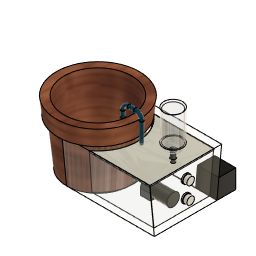
양액 만드는 화분 (Autodesk Fusion 360 design; units mm, degrees)
Autodesk Fusion 360 part; units mm, degrees
note: some values were not read from the file. Chosen so that the rebuilt part matches the saved one: which bodies a step acts on; which sketch regions a step uses; which face or edge a step refers to.
sketch "스케치1" plane through (0, 0, 0) normal (0, 0, 1) x (1, 0, 0)
  circle A0 through (55, 25, 50) (10, 50.9808, 50) (10, -0.9808, 50)
  circle A1 centre (25, 25) radius 25
sketch "스케치1 (curves 50 mm off its plane)" plane through (0, 0, 50) normal (0, 0, 1) x (1, 0, 0)
  circle A0 centre (25, 25) radius 30
loft "로프트1" add profiles "스케치1", "스케치1 (curves 50 mm off its plane)" section 1 section 2 makes body 1
shell "쉘1" thickness 3 removed faces 1 at (36.9822, 20.8839, 50) on bodies 1
sketch "스케치2" plane through (0, 0, 50) normal (0, 0, 1) x (-1, 0, 0)
  circle A0 centre (-25, -25) radius 26.985
  circle A1 centre (-25, -25) radius 30
  circle A2 centre (-25, -25) radius 33
  dimension "d2" = 3
sketch "스케치3" plane through (0, 0, 0) normal (0, 0, -1) x (1, 0, 0)
  circle A0 centre (25, -25) radius 25
  circle A1 centre (25, -25) radius 28
  dimension "d3" = 3
loft "로프트2" add profiles "스케치3", "스케치2" section 1 contours A0 | A1 section 2 contours A2 separate body makes body 2
shell "쉘2" thickness 3 removed faces 1 at (19.7673, 16.6449, 50) on bodies 2
sketch "스케치4" plane through (0, 0, 0) normal (0, 1, 0) x (1, 0, 0)
  line L0 (-8, -37) -> (-8, 0)
  line L1 (-8, -37) -> (58, -37)
  line L2 (58, -37) -> (58, 0)
  line L3 (58, 0) -> (-8, 0)
  constraint vertical L0
  constraint perpendicular L0 L1
  constraint perpendicular L1 L2
  constraint perpendicular L0 L3
extrude "돌출1" cut sketch "스케치4" along normal blind 75 and the other way blind 20 bodies 2
combine "결합1" operation add target body 1 tool bodies 2
sketch "스케치5" plane through (0, 0, 0) normal (0, 0, -1) x (1, 0, 0)
  circle A0 centre (25, -25) radius 25
  line L0 (25, 0) -> (95, 0)
  line L1 (95, 0) -> (95, -50)
  line L2 (95, -50) -> (25, -50)
  constraint coincident A0 L0.start
  constraint tangent A0 L0
  constraint horizontal L0
  constraint perpendicular L0 L1
  constraint coincident A0 L2.end
  constraint tangent A0 L2
  constraint perpendicular L1 L2
sketch "스케치6" plane through (0, 0, 50) normal (0, 0, 1) x (-1, 0, 0)
  circle A0 centre (-25, -25) radius 33
  circle A1 centre (-25, -25) radius 26.985
  line L0 (-25, -55) -> (-95, -55)
  line L1 (-95, -55) -> (-95, 5)
  line L2 (-95, 5) -> (-25, 5)
  circle A2 centre (-25, -25) radius 30
  constraint horizontal L0
  constraint perpendicular L0 L1
  constraint perpendicular L1 L2
  constraint concentric A0 A2
loft "로프트3" add profiles "스케치5", "스케치6" section 1 contours A0 L0 L1 L2 section 2 contours A0 L0 L2 A2 | A0 L0 L1 L2 picked at (-55.9441, -25) separate body makes body 3
sketch "스케치7" plane through (0, 0, 0) normal (0, 1, 0) x (1, 0, 0)
  line L0 (95, -50) -> (95, -37)
  line L1 (95, -37) -> (25, -37)
  line L2 (25, -37) -> (25, -50)
  line L3 (25, -50) -> (95, -50)
  constraint vertical L0
  constraint perpendicular L0 L1
  constraint perpendicular L1 L2
  constraint perpendicular L0 L3
extrude "돌출2" cut sketch "스케치7" along normal mid plane 210 bodies 3
shell "쉘3" thickness 3 removed faces 1 at (81.2007, 24.21, 37) on bodies 3
sketch "스케치8" plane through (0, 0, 3) normal (0, 0, 1) x (-1, 0, 0)
  line L0 (-92, -2.715) -> (-92, -47.285)
  line L1 (-92, -47.285) -> (-42.4675, -47.285)
  arc A0 (-42.4675, -2.715) -> (-42.4675, -47.285) centre (-25, -25) ccw
  line L2 (-42.4675, -2.715) -> (-92, -2.715)
sketch "스케치9" plane through (0, 0, 37) normal (0, 0, 1) x (-1, 0, 0)
  arc A0 (-43.6042, 0.685) -> (-43.6042, -50.685) centre (-25, -25) ccw
  line L0 (-43.6042, -50.685) -> (-92, -50.685)
  line L1 (-92, -50.685) -> (-92, 0.685)
  line L2 (-92, 0.685) -> (-43.6042, 0.685)
  line L3 (-25, 3.7) -> (-95, 3.7)
  line L4 (-95, 3.7) -> (-95, -53.7)
  line L5 (-95, -53.7) -> (-25, -53.7)
  arc A1 (-25, 3.7) -> (-25, -53.7) centre (-25, -25) ccw
loft "로프트4" add profiles "스케치8", "스케치9" section 1 section 2 contours A0 L0 L1 L2 separate body makes body 4
sketch "스케치10" plane through (0, 0, 0) normal (0, 1, 0) x (1, 0, 0)
  line L0 (92, -34) -> (92, -3)
  line L1 (92, -34) -> (43, -34)
  line L2 (43, -34) -> (41, -3)
  line L3 (41, -3) -> (92, -3)
  constraint vertical L0
  constraint perpendicular L0 L1
  constraint perpendicular L0 L3
extrude "돌출3" cut sketch "스케치10" along normal mid plane 180 bodies 4
combine "결합2" operation add target body 3 tool bodies 4
sketch "스케치11" plane through (0, 0, 37) normal (0, 0, 1) x (-1, 0, 0)
  line L0 (-25, 3.7) -> (-95, 3.7)
  line L1 (-95, 3.7) -> (-95, -53.7)
  line L2 (-95, -53.7) -> (-25, -53.7)
  arc A0 (-25, 3.7) -> (-25, -53.7) centre (-25, -25) ccw
  circle A1 centre (-85, -25) radius 1.5
  dimension "d58" = 3
  measures "d58" diameter of A1
extrude "돌출4" cut sketch "스케치11" against normal blind 6 contours A1 bodies 3
sketch "스케치12" plane through (0, 0, 37) normal (0, 0, 1) x (-1, 0, 0)
  circle A0 centre (-85, -25) radius 1.5
  line L0 (-25, 3.7) -> (-95, 3.7)
  line L1 (-95, 3.7) -> (-95, -53.7)
  line L2 (-95, -53.7) -> (-25, -53.7)
  arc A1 (-25, 3.7) -> (-25, -53.7) centre (-25, -25) ccw
  circle A2 centre (-85, -25) radius 2.5
  dimension "d59" = 5
  constraint concentric A0 A2
  measures "d59" diameter of A2
extrude "돌출5" add sketch "스케치12" against normal blind 3 separate body contours A0 makes body 5
extrude "돌출6" add sketch "스케치12" along normal blind 15 contours A0 | A2 bodies 5
sketch "스케치13" plane through (0, 0, 52) normal (0, 0, 1) x (-1, 0, 0)
  circle A0 centre (-85, -25) radius 2.5
  circle A1 centre (-85, -25) radius 7.5
  constraint concentric A0 A1
extrude "돌출7" add sketch "스케치13" along normal blind 30 separate body contours A0 | A1 makes body 6
fillet "모깎기1" radius 4 1 edges at (91.9925, 27.7121, 52) on bodies 6
sketch "스케치14" plane through (0, 0, 0) normal (1, 0, 0) x (0, 1, 0)
  circle A0 centre (25, 10.5) radius 7.5
  line L0 (32.5, 10.5) -> (32.5, 3)
  line L1 (17.5, 10.5) -> (17.5, 3)
  line L2 (17.5, 3) -> (32.5, 3)
  constraint coincident A0 L0.start
  constraint tangent A0 L0
  constraint vertical L0
  constraint coincident A0 L1.start
  constraint tangent A0 L1
  constraint vertical L1
  constraint perpendicular L0 L2
extrude "돌출8" add sketch "스케치14" along normal blind 92 and the other way blind -62 separate body makes body 7
extrude "돌출9" cut sketch "스케치14" along normal blind 92 and the other way blind -77 contours A0 L0 L2 | A0 L1 L2 bodies 7
sketch "스케치15" plane through (0, 0, 0) normal (0, 1, 0) x (1, 0, 0)
  line L0 (59.8497, -14.5) -> (59.8497, -50)
  line L1 (54.8497, -55) -> (49.8497, -55)
  line L2 (44.8497, -50) -> (44.8497, -45)
  arc A0 (44.8497, -50) -> (49.8497, -55) centre (49.8497, -50) ccw
  arc A1 (54.8497, -55) -> (59.8497, -50) centre (54.8497, -50) ccw
  arc A2 (61.8497, -12.5) -> (59.8497, -14.5) centre (61.8497, -14.5) ccw
  line L3 (61.8497, -12.5) -> (63.8497, -12.5)
  point P0 (59.8497, -12.5)
  point P1 (59.8497, -55)
  point P2 (44.8497, -55)
  dimension "d35" = 42.5
  dimension "d36" = 15
  dimension "d37" = 10
  dimension "d38" = 5
  dimension "d39" = 2
  dimension "d40" = 2
  constraint perpendicular L0 L1
  constraint perpendicular L1 L2
  constraint coincident P2 L1
  constraint coincident P2 L2
  constraint tangent L1 A0
  constraint tangent L2 A0
  constraint coincident P1 L0
  constraint coincident P1 L1
  constraint tangent L0 A1
  constraint tangent L1 A1
  constraint equal A0 A1
  constraint coincident P0 L0
  constraint tangent L0 A2
  measures "d35" distance of P0 P1
  measures "d36" distance of P1 P2
  measures "d37" distance of P2 L2.end
  measures "d38" radius of A0
  measures "d39" radius of A2
  measures "d40" distance of A2.start L3.end
pipe "파이프1" add diameter 3 wall 0.5 path "스케치15" along L3 A2 L0 A1 L1 A0 L2 separate body makes body 8
extrude "돌출10" cut 1 faces at (62, 22.5, 8) along direction (1, 0, 0) blind 2 on bodies 7 bodies 7
extrude "돌출11" cut 1 faces at (92, 22.8, 8.5012) along direction (-1, 0, 0) blind 2 on bodies 7 bodies 7
move_body "이동1" bodies 8 to x (1, 0, 0) y (0, 1, 0) z (0, 0, 1) at (0, 25, 0)
sketch "스케치16" plane through (95, 0, 0) normal (1, 0, 0) x (0, 1, 0)
  line L0 (53.7, 37) -> (-3.7, 37)
  line L1 (-3.7, 37) -> (0, 0)
  line L2 (0, 0) -> (50, 0)
  line L3 (50, 0) -> (53.7, 37)
  circle A0 centre (25, 9.25) radius 3.5
  circle A1 centre (25, 9.25) radius 3
  circle A2 centre (25, 27.75) radius 3.5
  circle A3 centre (25, 27.75) radius 3
  dimension "d49" = 7
  dimension "d50" = 6
  constraint concentric A0 A1
  measures "d49" diameter of A0
  measures "d50" diameter of A1
extrude "돌출12" add sketch "스케치16" along normal blind 1 separate body contours A0 | A1 | A2 | A3 makes body 9 at (95, 23.9489, 28.2562) makes body 10 at (95, 23.3018, 10.1706)
extrude "돌출13" add sketch "스케치16" along normal blind 4 contours A1 | A3 bodies 9 10
move_body "이동2" bodies 10 to x (1, 0, 0) y (0, 1, 0) z (0, 0, 1) at (0, 0, 5)
sketch "스케치17" plane through (0, 0, 52) normal (0, 0, 1) x (-1, 0, 0)
  circle A0 centre (-85, -25) radius 2.5
  circle A1 centre (-85, -25) radius 2
  dimension "d55" = -0.5
extrude "돌출14" cut sketch "스케치17" against normal blind 15 bodies 5
extrude "돌출15" cut 1 faces at (85.9581, 25.5552, 52) along direction (0, 0, -1) blind 5 on bodies 5 bodies 5
delete_face "면 삭제1" 1 faces at (86.592, 17.6895, 55.6198) on bodies 6
move_body "이동3" bodies 6 to x (1, 0, 0) y (0, 1, 0) z (0, 0, 1) at (0, 0, -5)
fillet "모깎기2" radius 5.5 1 edges at (91.9925, 22.2879, 47) on bodies 6
extrude "돌출16" cut 1 faces at (84.435, 25.228, 47) along direction (0, 0, -1) blind 5 on bodies 5 bodies 5
move_body "이동4" bodies 6 to x (1, 0, 0) y (0, 1, 0) z (0, 0, 1) at (0, 0, -5)
shell "쉘4" thickness 1 removed faces 1 at (86.7678, 24.8544, 72) on bodies 6
extrude "돌출17" cut 1 faces at (86.386, 25.2526, 43) along direction (0, 0, -1) blind 11 on bodies 6 bodies 6
sketch "스케치18" plane through (0, 0, 72) normal (0, 0, 1) x (-1, 0, 0)
  circle A0 centre (-85, -25) radius 6.5
  circle A1 centre (-85, -25) radius 7.5
extrude "돌출18" add sketch "스케치18" against normal blind 1 contours A0 bodies 6
sketch "스케치19" plane through (0, 0, 37) normal (0, 0, 1) x (-1, 0, 0)
  circle A0 centre (-85, -25) radius 1.5
  line L0 (-25, 3.7) -> (-95, 3.7)
  line L1 (-95, 3.7) -> (-95, -53.7)
  line L2 (-95, -53.7) -> (-25, -53.7)
  arc A1 (-25, 3.7) -> (-25, -53.7) centre (-25, -25) ccw
  arc A2 (-43.558, 0.7) -> (-43.558, -50.7) centre (-25, -25) ccw
  line L3 (-92, -50.7) -> (-43.558, -50.7)
  line L4 (-92, 0.7) -> (-92, -50.7)
  line L5 (-43.558, 0.7) -> (-92, 0.7)
  dimension "d71" = -3
extrude "돌출19" add sketch "스케치19" against normal blind 1 separate body contours A0 | A2 L3 L4 L5 makes body 11
move_body "이동5" bodies 11 to x (1, 0, 0) y (0, 1, 0) z (0, 0, 1) at (0, 0, -3)
sketch "스케치20" plane through (90, 0, 0) normal (1, 0, 0) x (0, 1, 0)
  circle A0 centre (25, 10.5) radius 7.5
  line L0 (25, 10.5) -> (25, 3)
  circle A1 centre (25, 8) radius 5
  line L1 (20, 8) -> (20, 3)
  line L2 (20, 3) -> (30, 3)
  line L3 (30, 3) -> (30, 8)
  line L4 (20, 3) -> (17.5, 3)
  line L5 (25, 10.5) -> (17.5, 10.5)
  line L6 (17.5, 10.5) -> (17.5, 3)
  line L7 (25, 10.5) -> (32.5, 10.5)
  line L8 (32.5, 10.5) -> (32.5, 3)
  line L9 (32.5, 3) -> (30, 3)
  dimension "d74" = 10
  dimension "d81" = 5
  dimension "d82" = 10
  dimension "d83" = 2.5
  constraint coincident A0.centre L0.start
  constraint coincident A0 L0.end
  constraint vertical L0
  constraint coincident L0.end A1
  constraint coincident A1 L1.start
  constraint parallel L0 L1
  constraint perpendicular L0 L2
  constraint perpendicular L2 L3
  constraint perpendicular L1 L4
  constraint coincident A0 L5.end
  constraint perpendicular L0 L5
  constraint coincident A0 L7.end
  constraint perpendicular L0 L7
  constraint tangent A0 L8
  constraint perpendicular L8 L9
  measures "d74" diameter of A1
  measures "d81" distance of L1.start L1.end
  measures "d82" distance of L1.end L2.end
  measures "d83" distance of L1.end L4.end
extrude "돌출20" cut sketch "스케치20" against normal blind 26 contours A0 A1 L5 L7 | A0 A1 L3 L7 | A0 A1 L1 L5 | A0 A1 L3 | A0 A1 L1 bodies 7
extrude "돌출21" cut 1 faces at (90, 26.8176, 7.0783) along direction (-1, 0, 0) blind 5 on bodies 7 bodies 7
extrude "돌출22" cut 2 faces at (77, 18.7097, 4.7628) (77, 31.2903, 4.7628) along direction (-1, 0, 0) blind 5 on bodies 7 bodies 7
extrude "돌출23" cut sketch "스케치20" against normal blind 27 contours A0 L3 L8 L9 | A0 L1 L4 L6 bodies 7
extrude "돌출24" add sketch "스케치20" along normal blind -26 and the other way blind 18 contours A0 A1 L3 | A0 A1 L1 bodies 7
sketch "스케치21" plane through (0, 0, 0) normal (0, 1, 0) x (1, 0, 0)
  line L0 (55.0005, -25.1034) -> (63.5375, -25.1034)
  constraint horizontal L0
split "분할1" by curves path "스케치21" along L0 bodies 8 makes body 12 at (60.1102, 26.4772, 41.7011)
move_body "이동6" bodies 8 to x (1, 0, 0) y (0, 1, 0) z (0, 0, 1) at (0, 0, -3)
extrude "돌출25" add 1 faces at (58.5406, 24.8006, 22.1034) along direction (0, 0, 1) blind 3 on bodies 8 bodies 8 12
sketch "스케치22" plane through (95, 0, 0) normal (1, 0, 0) x (0, 1, 0)
  line L0 (53.7, 37) -> (-3.7, 37)
  line L1 (-3.7, 37) -> (0, 0)
  line L2 (0, 0) -> (50, 0)
  line L3 (50, 0) -> (53.7, 37)
  line L4 (50, 0) -> (65, 0)
  line L5 (65, 0) -> (65, 15)
  line L6 (65, 15) -> (50, 15)
  line L7 (50, 15) -> (50, 0)
  dimension "d92" = 15
  dimension "d93" = 15
  constraint horizontal L4
  constraint vertical L5
  constraint horizontal L6
  constraint vertical L7
  constraint coincident L2.end L3.start
  measures "d92" distance of L2.end L4.end
  measures "d93" distance of L2.end L6.end
extrude "돌출26" add sketch "스케치22" against normal blind 17 separate body contours L3 L4 L5 L6 makes body 13
